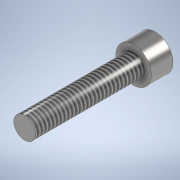
# Autodesk Inventor part: TornilloM4X20mm
Saved by Autodesk Inventor 2021.5 (Build 255421000, 421)
## iProperties
Created: 2024-11-29
Part Number: TornilloM4X20mm
Material: Acero inoxidable
Document SubType Name: Modeling
Designer: Joho_
Mass: 2.9062 g
Surface Area: 4.23375 cm^2
Volume: 0.363275 cm^3
Density: 8 g/cm^3
Appearance: Semipulido
Author: Joho_
Autodesk Inventor part; units mm, degrees
ref_plane "YZ Plane" through (0, 0, 0) normal (1, 0, 0) x (0, 1, 0)
ref_plane "XZ Plane" through (0, 0, 0) normal (0, 1, 0) x (-1, 0, 0)
ref_plane "XY Plane" through (0, 0, 0) normal (0, 0, 1) x (1, 0, 0)
sketch "Boceto1" plane through (0, 0, 0) normal (0, 0, 1) x (1, 0, 0)
  circle A0 centre (0, 0) radius 2
  circle A1 centre (0, 0) radius 3.25
  dimension "d0" = 4
  dimension "d1" = 6.5
  constraints: 3 coincident, 2 centre point
  measures "d0" diameter of A0
  measures "d1" diameter of A1
extrude "Extrusión1" add sketch "Boceto1" along normal blind 20 contours A0
extrude "Extrusión2" add sketch "Boceto1" against normal blind 4 contours A0 | A1
sketch "Boceto2" plane through (0, 0, -4) normal (0, 0, -1) x (-1, 0, 0)
  line L0 (2, 0) -> (1, -1.7321)
  line L1 (1, -1.7321) -> (-1, -1.7321)
  line L2 (-1, -1.7321) -> (-2, 0)
  line L3 (-2, 0) -> (-1, 1.7321)
  line L4 (-1, 1.7321) -> (1, 1.7321)
  line L5 (1, 1.7321) -> (2, 0)
  point P0 (0, 0)
  point P1 (0, 0)
  dimension "d6" = 4
  constraints: 12 end point, 1 coincident, 13 other
  measures "d6" distance of L0.start L2.end
extrude "Extrusión3" cut sketch "Boceto2" against normal blind 2
thread "Rosca1" size "M4x0.7" class "6g" standard "ANSI Metric M Profile" full length
